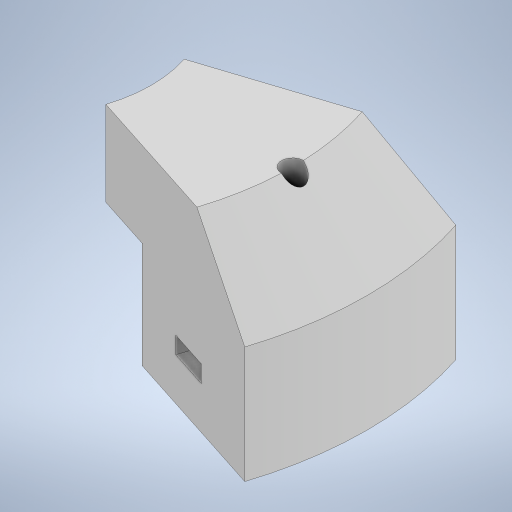
# Autodesk Inventor part: Деталь1
Saved by Autodesk Inventor 2023 (Build 270158000, 158)
## iProperties
Created: 2025-02-05
Part Number: Деталь1
Material: Типовые
Document SubType Name: Modeling
Designer: baranovaem
Density: 1 g/cm^3
Appearance: По умолчанию
Author: baranovaem
Autodesk Inventor part; units mm, degrees
ref_plane "YZ Plane" through (0, 0, 0) normal (1, 0, 0) x (0, 1, 0)
ref_plane "XZ Plane" through (0, 0, 0) normal (0, 1, 0) x (-1, 0, 0)
ref_plane "XY Plane" through (0, 0, 0) normal (0, 0, 1) x (1, 0, 0)
sketch "Эскиз3" plane through (0, 0, 0) normal (0, 0, 1) x (1, 0, 0)
  line L0 (26, 0) -> (48.5118, 0)
  line L1 (48.5118, 0) -> (48.5118, 16.4882)
  line L2 (26, 15) -> (18, 15)
  line L3 (18, 15) -> (18, 27)
  line L4 (18, 27) -> (38, 27)
  line L5 (38, 27) -> (48.5118, 16.4882)
  line L6 (38, 27) -> (52.866, 27) construction
  line L7 (26, 15) -> (26, 0)
  dimension "d18" = 14.866
  dimension "d19" = 45
  dimension "d20" = 20
  dimension "d25" = 8
  constraints: 16 end point, 3 horizontal, 2 perpendicular, 1 equal length, 1 parallel
  measures "d18" distance of L4.end L1.end
  measures "d19" angle of L5 L6
  measures "d20" distance of L3.end L4.end
  measures "d25" distance of L2.end L2.start
sketch "Эскиз4" plane through (0, 0, 0) normal (0, 1, 0) x (-1, 0, 0)
  arc A0 (-24.7386, 8) -> (-24.7386, -8) centre (0, 0) ccw
  dimension "d31" = 26
  constraints: 2 point on circle, 1 centre point
  measures "d31" radius of A0
sweep "Сдвиг1" add profiles "Эскиз3" path "Эскиз4"
sketch "Эскиз5" plane through (0, 0, 0) normal (0, -1, 0) x (1, 0, 0)
  arc A0 (36.1565, 11.6923) -> (36.1565, -11.6923) centre (0, 0) ccw projected
  circle A1 centre (38, 0) radius 1.575
  point P0 (0, 0)
  dimension "d27" = 3.15
  constraints: 1 centre point, 1 point on circle
  measures "d27" diameter of A1
extrude "Выдавливание2" cut sketch "Эскиз5" against normal up to surface (27 mm away)
sketch "Эскиз7" plane through (46.1583, 0, 14.9267) normal (-0.3076923, 0, 0.9514859) x (0.9514859, 0, 0.3076923)
  line L0 (-13.9304, 0) -> (-13.9304, 27) projected
  line L1 (-10.7804, 0) -> (-10.7804, 25.4984) projected
  line L2 (-13.9304, 0) -> (-10.7804, 0)
  line L3 (-12.3554, 12.4) -> (-12.3554, 0) construction
  line L4 (-22.5118, 0) -> (0, 0) projected
  line L5 (-15.1554, 8.4) -> (-9.5554, 8.4)
  line L6 (-9.5554, 8.4) -> (-9.5554, 6)
  line L7 (-9.5554, 6) -> (-15.1554, 6)
  line L8 (-15.1554, 6) -> (-15.1554, 8.4)
  line L9 (-9.5554, 6) -> (-15.1554, 8.4) construction
  point P0 (-48.5118, 0)
  point P1 (-12.3554, 7.2)
  dimension "d35" = 5.6
  dimension "d36" = 2.4
  dimension "d37" = 1.575
  dimension "d38" = 6
  constraints: 14 end point, 2 parallel, 2 perpendicular, 2 point on line, 1 horizontal, 1 midpoint
  measures "d35" distance of L6.end L7.end
  measures "d36" distance of L5.end L6.end
  measures "d37" distance between parallel lines of L1 L3
  measures "d38" distance between parallel lines of L4 L7
extrude "Выдавливание3" cut sketch "Эскиз7" against normal blind 14 contours L7 L8 L5 L0 | L0 L5 L1 L7 | L1 L5 L6 L7
